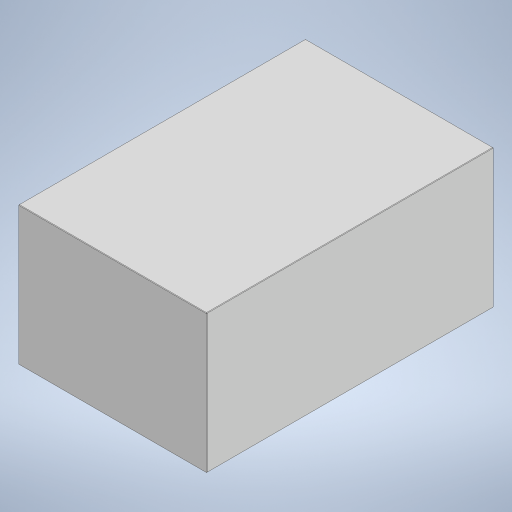
# Autodesk Inventor part: box elektronik
Saved by Autodesk Inventor 2023 (Build 270158000, 158)
## iProperties
Created: 2023-09-20
Part Number: box elektronik
Material: Generic
Document SubType Name: Modeling
Designer: sigit
Density: 1 g/cm^3
Appearance: Default
Author: sigit
Autodesk Inventor part; units mm, degrees
ref_plane "YZ Plane" through (0, 0, 0) normal (1, 0, 0) x (0, 1, 0)
ref_plane "XZ Plane" through (0, 0, 0) normal (0, 1, 0) x (-1, 0, 0)
ref_plane "XY Plane" through (0, 0, 0) normal (0, 0, 1) x (1, 0, 0)
sketch "Sketch1" plane through (0, 0, 0) normal (0, 1, 0) x (-1, 0, 0)
  line L0 (0, 0) -> (190, 0)
  line L1 (190, 0) -> (190, -290)
  line L2 (190, -290) -> (0, -290)
  line L3 (0, -290) -> (0, 0)
  dimension "d0" = 190
  dimension "d1" = 290
  constraints: 8 end point, 2 parallel, 1 horizontal, 1 perpendicular
  measures "d0" distance of L1.end L2.end
  measures "d1" distance of L0.end L1.end
extrude "Extrusion1" add sketch "Sketch1" along normal blind 140
fillet "Fillet1" radius 0.5 12 edges at (-95, 140, -290) (-95, 0, -290) (-190, 70, -290) (-190, 140, -145) (-190, 0, -145) (-190, 70, 0) (-95, 140, 0) (-95, 0, 0) (0, 70, 0) (0, 140, -145) (0, 70, -290) (0, 0, -145)
body "Solid1"
